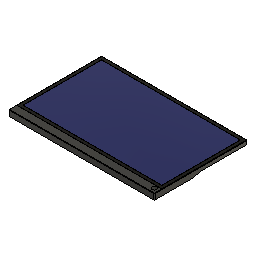
Monitor Frame3 v19 (Autodesk Fusion 360 archive; units mm, degrees)
design "TC Monitor"
Autodesk Fusion 360 part; units mm, degrees
note: some values were not read from the file. Chosen so that the rebuilt part matches the saved one: which pieces of a blend or face edit are solid.
sketch "Sketch1" plane through (0, 0, 0) normal (0, 0, 1) x (1, 0, 0)
  line L0 (0, 0) -> (373.8, 0)
  line L1 (373.8, 0) -> (373.8, 238.3)
  line L2 (373.8, 238.3) -> (0, 238.3)
  line L3 (0, 238.3) -> (0, 0)
  circle A0 centre (361.8, 12) radius 6
  line L4 (1, 237.3) -> (372.8, 237.3)
  line L5 (372.8, 237.3) -> (372.8, 20)
  line L6 (372.8, 20) -> (1, 20)
  line L7 (1, 20) -> (1, 237.3)
  line L8 (9, 229.3) -> (364.8, 229.3)
  line L9 (364.8, 229.3) -> (364.8, 28)
  line L10 (364.8, 28) -> (9, 28)
  line L11 (9, 28) -> (9, 229.3)
  dimension "d1" = 373.8
  dimension "d2" = 238.3
  dimension "d3" = 12
  dimension "d4" = 12
  dimension "d5" = 12
  dimension "d6" = 1
  dimension "d7" = 1
  dimension "d8" = 1
  dimension "d9" = 20
  dimension "d10" = 8
  constraint horizontal L0
  constraint vertical L1
  constraint horizontal L2
  constraint vertical L3
  constraint coincident L0.start L3.end
  constraint horizontal L4
  constraint vertical L5
  constraint horizontal L6
  constraint vertical L7
  measures "d1" distance of L0.start L0.end
  measures "d2" distance of L0.start L2.end
  measures "d3" distance of L1 A0.centre
  measures "d4" distance of L0 A0.centre
  measures "d5" diameter of A0
  measures "d6" distance of L3 L7
  measures "d7" distance of L2 L4
  measures "d8" distance of L1 L5
  measures "d9" distance of L0 L6
extrude "Extrude1" add sketch "Sketch1" against normal blind 15 contours L0 L1 L2 L3 | L4 L5 L6 L7 | L8 L9 L10 L11
extrude "Extrude2" cut sketch "Sketch1" against normal blind 0.5 contours L4 L5 L6 L7
sketch "Sketch2" plane through (0, 0, -15) normal (0, 0, -1) x (1, 0, 0)
  circle A0 centre (361.8, -12) radius 6
  line L0 (0, 0) -> (0, -238.3)
  line L1 (0, -238.3) -> (373.8, -238.3)
  line L2 (373.8, -238.3) -> (373.8, 0)
  line L3 (373.8, 0) -> (0, 0)
  line L4 (373.8, -119.15) -> (0, -119.15)
  constraint midpoint L2 L4.start
  constraint midpoint L0 L4.end
extrude "Extrude3" cut sketch "Sketch2" against normal blind 5 contours L0 L1 L2 L4
chamfer "Chamfer1" distance 20 distance2 5 1 edges at (186.9, 119.15, -15) measured on face at (118.6889, 44.3062, -15)
fillet "Fillet2" radius 2 4 edges at (0, 0, -7.5) (373.8, 0, -7.5) (373.8, 238.3, -5) (0, 238.3, -5)
fillet "Fillet1" radius 1 4 edges at (0, 119.15, 0) (186.9, 0, 0) (373.8, 119.15, 0) (186.9, 238.3, 0)
sketch "Sketch3" plane through (0, 0, -10) normal (0, 0, -1) x (1, 0, 0)
  arc A0 (0, -236.3) -> (2, -238.3) centre (2, -236.3) ccw
  line L0 (2, -238.3) -> (371.8, -238.3)
  arc A1 (371.8, -238.3) -> (373.8, -236.3) centre (371.8, -236.3) ccw
  line L1 (373.8, -236.3) -> (373.8, -119.15)
  line L2 (373.8, -119.15) -> (0, -119.15)
  line L3 (0, -119.15) -> (0, -236.3)
  circle A2 centre (307.4, -208.3) radius 1.5
  circle A3 centre (66.4, -208.3) radius 1.5
  dimension "d21" = 3
  dimension "d22" = 3
  dimension "d23" = 30
  dimension "d24" = 30
  dimension "d25" = 241
  dimension "d26" = 373.8
  dimension "d27" = 66.4
  measures "d21" diameter of A2
  measures "d22" diameter of A3
  measures "d23" distance of L0 A2.centre
  measures "d24" distance of L0 A3.centre
  measures "d25" distance of A2.centre A3.centre
  measures "d26" distance of L1 L3
  measures "d27" distance of L1 A2.centre
extrude "Extrude4" cut sketch "Sketch3" against normal blind 5 contours A2 | A3
equation "d7 = d6"
equation "d8 = d6"
equation "d22 = d21"
equation "d24 = d23"
equation "d27 = ( 373.80 mm - d25 ) / 2"

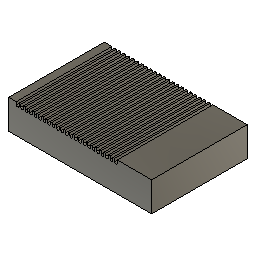
design "Mini_PC"
Autodesk Fusion 360 part; units mm, degrees
sketch "Sketch1" plane through (0, 0, 0) normal (0, 0, 1) x (1, 0, 0)
  line L0 (0, 0) -> (160, 0)
  line L1 (160, 0) -> (160, 107)
  line L2 (160, 107) -> (0, 107)
  line L3 (0, 107) -> (0, 0)
  dimension "d1" = 160
  dimension "d2" = 107
  constraint horizontal L0
  constraint vertical L1
  constraint horizontal L2
  constraint vertical L3
  constraint coincident L0.start L3.end
  measures "d1" distance of L0.start L0.end
  measures "d2" distance of L0.start L2.end
extrude "Extrude1" add sketch "Sketch1" along normal blind 33
sketch "Sketch2" plane through (0, 0, 0) normal (0, -1, 0) x (1, 0, 0)
  line L0 (0, 0) -> (160, 0)
  line L1 (160, 0) -> (160, 33)
  line L2 (160, 33) -> (0, 33)
  line L3 (0, 33) -> (0, 0)
  line L4 (11.5, 30) -> (11.5, 37.085)
  arc A0 (11.5, 37.085) -> (8.5, 37.085) centre (10, 37.085) ccw
  line L5 (8.5, 37.085) -> (8.5, 30)
  arc A1 (8.5, 30) -> (11.5, 30) centre (10, 30) ccw
  line L6 (10, 30) -> (10, 37.085) construction
  line L7 (16.5, 30) -> (16.5, 37.085)
  arc A2 (13.5, 30) -> (16.5, 30) centre (15, 30) ccw
  line L8 (13.5, 37.085) -> (13.5, 30)
  arc A3 (16.5, 37.085) -> (13.5, 37.085) centre (15, 37.085) ccw
  line L9 (21.5, 30) -> (21.5, 37.085)
  arc A4 (18.5, 30) -> (21.5, 30) centre (20, 30) ccw
  line L10 (18.5, 37.085) -> (18.5, 30)
  arc A5 (21.5, 37.085) -> (18.5, 37.085) centre (20, 37.085) ccw
  line L11 (26.5, 30) -> (26.5, 37.085)
  arc A6 (23.5, 30) -> (26.5, 30) centre (25, 30) ccw
  line L12 (23.5, 37.085) -> (23.5, 30)
  arc A7 (26.5, 37.085) -> (23.5, 37.085) centre (25, 37.085) ccw
  line L13 (31.5, 30) -> (31.5, 37.085)
  arc A8 (28.5, 30) -> (31.5, 30) centre (30, 30) ccw
  line L14 (28.5, 37.085) -> (28.5, 30)
  arc A9 (31.5, 37.085) -> (28.5, 37.085) centre (30, 37.085) ccw
  line L15 (36.5, 30) -> (36.5, 37.085)
  arc A10 (33.5, 30) -> (36.5, 30) centre (35, 30) ccw
  line L16 (33.5, 37.085) -> (33.5, 30)
  arc A11 (36.5, 37.085) -> (33.5, 37.085) centre (35, 37.085) ccw
  line L17 (41.5, 30) -> (41.5, 37.085)
  arc A12 (38.5, 30) -> (41.5, 30) centre (40, 30) ccw
  line L18 (38.5, 37.085) -> (38.5, 30)
  arc A13 (41.5, 37.085) -> (38.5, 37.085) centre (40, 37.085) ccw
  line L19 (46.5, 30) -> (46.5, 37.085)
  arc A14 (43.5, 30) -> (46.5, 30) centre (45, 30) ccw
  line L20 (43.5, 37.085) -> (43.5, 30)
  arc A15 (46.5, 37.085) -> (43.5, 37.085) centre (45, 37.085) ccw
  line L21 (51.5, 30) -> (51.5, 37.085)
  arc A16 (48.5, 30) -> (51.5, 30) centre (50, 30) ccw
  line L22 (48.5, 37.085) -> (48.5, 30)
  arc A17 (51.5, 37.085) -> (48.5, 37.085) centre (50, 37.085) ccw
  line L23 (56.5, 30) -> (56.5, 37.085)
  arc A18 (53.5, 30) -> (56.5, 30) centre (55, 30) ccw
  line L24 (53.5, 37.085) -> (53.5, 30)
  arc A19 (56.5, 37.085) -> (53.5, 37.085) centre (55, 37.085) ccw
  line L25 (61.5, 30) -> (61.5, 37.085)
  arc A20 (58.5, 30) -> (61.5, 30) centre (60, 30) ccw
  line L26 (58.5, 37.085) -> (58.5, 30)
  arc A21 (61.5, 37.085) -> (58.5, 37.085) centre (60, 37.085) ccw
  line L27 (66.5, 30) -> (66.5, 37.085)
  arc A22 (63.5, 30) -> (66.5, 30) centre (65, 30) ccw
  line L28 (63.5, 37.085) -> (63.5, 30)
  arc A23 (66.5, 37.085) -> (63.5, 37.085) centre (65, 37.085) ccw
  line L29 (71.5, 30) -> (71.5, 37.085)
  arc A24 (68.5, 30) -> (71.5, 30) centre (70, 30) ccw
  line L30 (68.5, 37.085) -> (68.5, 30)
  arc A25 (71.5, 37.085) -> (68.5, 37.085) centre (70, 37.085) ccw
  line L31 (76.5, 30) -> (76.5, 37.085)
  arc A26 (73.5, 30) -> (76.5, 30) centre (75, 30) ccw
  line L32 (73.5, 37.085) -> (73.5, 30)
  arc A27 (76.5, 37.085) -> (73.5, 37.085) centre (75, 37.085) ccw
  line L33 (81.5, 30) -> (81.5, 37.085)
  arc A28 (78.5, 30) -> (81.5, 30) centre (80, 30) ccw
  line L34 (78.5, 37.085) -> (78.5, 30)
  arc A29 (81.5, 37.085) -> (78.5, 37.085) centre (80, 37.085) ccw
  line L35 (86.5, 30) -> (86.5, 37.085)
  arc A30 (83.5, 30) -> (86.5, 30) centre (85, 30) ccw
  line L36 (83.5, 37.085) -> (83.5, 30)
  arc A31 (86.5, 37.085) -> (83.5, 37.085) centre (85, 37.085) ccw
  line L37 (91.5, 30) -> (91.5, 37.085)
  arc A32 (88.5, 30) -> (91.5, 30) centre (90, 30) ccw
  line L38 (88.5, 37.085) -> (88.5, 30)
  arc A33 (91.5, 37.085) -> (88.5, 37.085) centre (90, 37.085) ccw
  line L39 (96.5, 30) -> (96.5, 37.085)
  arc A34 (93.5, 30) -> (96.5, 30) centre (95, 30) ccw
  line L40 (93.5, 37.085) -> (93.5, 30)
  arc A35 (96.5, 37.085) -> (93.5, 37.085) centre (95, 37.085) ccw
  line L41 (101.5, 30) -> (101.5, 37.085)
  arc A36 (98.5, 30) -> (101.5, 30) centre (100, 30) ccw
  line L42 (98.5, 37.085) -> (98.5, 30)
  arc A37 (101.5, 37.085) -> (98.5, 37.085) centre (100, 37.085) ccw
  line L43 (106.5, 30) -> (106.5, 37.085)
  arc A38 (103.5, 30) -> (106.5, 30) centre (105, 30) ccw
  line L44 (103.5, 37.085) -> (103.5, 30)
  arc A39 (106.5, 37.085) -> (103.5, 37.085) centre (105, 37.085) ccw
  line L45 (111.5, 30) -> (111.5, 37.085)
  arc A40 (108.5, 30) -> (111.5, 30) centre (110, 30) ccw
  line L46 (108.5, 37.085) -> (108.5, 30)
  arc A41 (111.5, 37.085) -> (108.5, 37.085) centre (110, 37.085) ccw
  line L47 (116.5, 30) -> (116.5, 37.085)
  arc A42 (113.5, 30) -> (116.5, 30) centre (115, 30) ccw
  line L48 (113.5, 37.085) -> (113.5, 30)
  arc A43 (116.5, 37.085) -> (113.5, 37.085) centre (115, 37.085) ccw
  line L49 (121.5, 30) -> (121.5, 37.085)
  arc A44 (118.5, 30) -> (121.5, 30) centre (120, 30) ccw
  line L50 (118.5, 37.085) -> (118.5, 30)
  arc A45 (121.5, 37.085) -> (118.5, 37.085) centre (120, 37.085) ccw
  dimension "d5" = 3
  dimension "d8" = 110
  dimension "d9" = 0
  constraint tangent L4 A0
  constraint tangent A0 L5
  constraint parallel L4 L5
  constraint tangent L5 A1
  constraint tangent L4 A1
  constraint perpendicular L2 L6
  measures "d5" diameter of A0
extrude "Extrude2" cut sketch "Sketch2" against normal through all contours L2 L4 L5 A1 | L2 L49 A44 L50 | L2 L49 L50 A45 | L2 L7 A2 L8 | L2 L47 A42 L48 | L2 L47 L48 A43 | L2 L9 A4 L10 | L2 L45 A40 L46 | L2 L45 L46 A41 | L2 L11 A6 L12 | L2 L43 A38 L44 | L2 L43 L44 A39 | L2 L13 A8 L14 | L2 L41 A36 L42 | L2 L41 L42 A37 | L2 L15 A10 L16 | L2 L39 A34 L40 | L2 L39 L40 A35 | L2 L17 A12 L18 | L2 L37 A32 L38 | L2 L19 A14 L20 | L2 L35 A30 L36 | L2 L21 A16 L22 | L2 L33 A28 L34 | L2 L23 A18 L24 | L2 L31 A26 L32 | L2 L25 A20 L26 | L2 L29 A24 L30 | L2 L27 A22 L28
